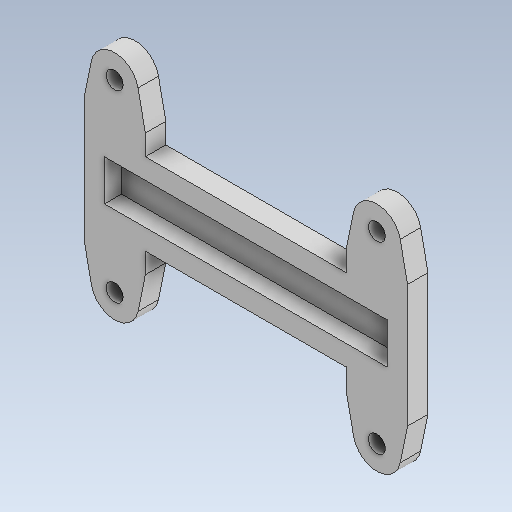
# Autodesk Inventor part: アーム下板
Saved by Autodesk Inventor 2020 (Build 240168000, 168)
## iProperties
Created: 2020-01-11
Part Number: アーム下板
Material: 一般
Document SubType Name: Modeling
Designer: tanjihayato
Density: 1 g/cm^3
Appearance: 既定
Mass: 2.01957 g
Surface Area: 26.5627 cm^2
Volume: 2.01957 cm^3
Author: tanjihayato
Autodesk Inventor part; units mm, degrees
ref_plane "YZ Plane" through (0, 0, 0) normal (1, 0, 0) x (0, 1, 0)
ref_plane "XZ Plane" through (0, 0, 0) normal (0, 1, 0) x (-1, 0, 0)
ref_plane "XY Plane" through (0, 0, 0) normal (0, 0, 1) x (1, 0, 0)
sketch "スケッチ1" plane through (0, 0, 0) normal (0, 0, 1) x (1, 0, 0)
  circle A0 centre (50.4, -4.5) radius 1.5
  circle A1 centre (50.4, -59) radius 1.5
  circle A2 centre (50.4, -86) radius 1.5
  circle A3 centre (50.4, -173.5) radius 1.5
  circle A4 centre (30.9, -4.5) radius 1.5
  circle A5 centre (30.9, -173.5) radius 1.5
  circle A6 centre (75.4, -4.5) radius 1.5
  circle A7 centre (75.4, -173.5) radius 1.5
  line L0 (38.1151, -78.5) -> (38.1151, -81.5)
  arc A8 (36.0151, -81.5) -> (38.1151, -81.5) centre (37.0651, -81.5) ccw
  line L1 (36.0151, -81.5) -> (25.2151, -81.5)
  arc A9 (23.1151, -81.5) -> (25.2151, -81.5) centre (24.1651, -81.5) ccw
  line L2 (23.1151, -81.5) -> (23.1151, -78.5)
  arc A10 (25.2151, -78.5) -> (23.1151, -78.5) centre (24.1651, -78.5) ccw
  line L3 (25.2151, -78.5) -> (36.0151, -78.5)
  arc A11 (38.1151, -78.5) -> (36.0151, -78.5) centre (37.0651, -78.5) ccw
  line L4 (-15.3701, -66.5) -> (-15.3701, -63.5)
  arc A12 (-13.2701, -63.5) -> (-15.3701, -63.5) centre (-14.3201, -63.5) ccw
  line L5 (-13.2701, -63.5) -> (-2.4701, -63.5)
  arc A13 (-0.3701, -63.5) -> (-2.4701, -63.5) centre (-1.4201, -63.5) ccw
  line L6 (-0.3701, -63.5) -> (-0.3701, -66.5)
  arc A14 (-2.4701, -66.5) -> (-0.3701, -66.5) centre (-1.4201, -66.5) ccw
  line L7 (-2.4701, -66.5) -> (-13.2701, -66.5)
  arc A15 (-15.3701, -66.5) -> (-13.2701, -66.5) centre (-14.3201, -66.5) ccw
  line L8 (-0.3701, -78.5) -> (-0.3701, -81.5)
  arc A16 (-2.4701, -81.5) -> (-0.3701, -81.5) centre (-1.4201, -81.5) ccw
  line L9 (-2.4701, -81.5) -> (-13.2701, -81.5)
  arc A17 (-15.3701, -81.5) -> (-13.2701, -81.5) centre (-14.3201, -81.5) ccw
  line L10 (-15.3701, -81.5) -> (-15.3701, -78.5)
  arc A18 (-13.2701, -78.5) -> (-15.3701, -78.5) centre (-14.3201, -78.5) ccw
  line L11 (-13.2701, -78.5) -> (-2.4701, -78.5)
  arc A19 (-0.3701, -78.5) -> (-2.4701, -78.5) centre (-1.4201, -78.5) ccw
  line L12 (23.1151, -66.5) -> (23.1151, -63.5)
  arc A20 (25.2151, -63.5) -> (23.1151, -63.5) centre (24.1651, -63.5) ccw
  line L13 (25.2151, -63.5) -> (36.0151, -63.5)
  arc A21 (38.1151, -63.5) -> (36.0151, -63.5) centre (37.0651, -63.5) ccw
  line L14 (38.1151, -63.5) -> (38.1151, -66.5)
  arc A22 (36.0151, -66.5) -> (38.1151, -66.5) centre (37.0651, -66.5) ccw
  line L15 (36.0151, -66.5) -> (25.2151, -66.5)
  arc A23 (23.1151, -66.5) -> (25.2151, -66.5) centre (24.1651, -66.5) ccw
  line L16 (-108.585, -50) -> (-111.585, -50)
  line L17 (-111.585, -50) -> (-111.585, -128)
  line L18 (-111.585, -128) -> (-108.585, -128)
  arc A24 (-108.585, -130.1) -> (-108.585, -128) centre (-108.585, -129.05) ccw
  line L19 (-108.585, -130.1) -> (-108.585, -140.9)
  arc A25 (-108.585, -143) -> (-108.585, -140.9) centre (-108.585, -141.95) ccw
  line L20 (-108.585, -143) -> (-111.585, -143)
  line L21 (-111.585, -143) -> (-111.585, -168)
  line L22 (-111.585, -168) -> (-108.585, -168)
  line L23 (-108.585, -168) -> (-108.585, -165)
  arc A26 (-106.485, -165) -> (-108.585, -165) centre (-107.535, -165) ccw
  line L24 (-106.485, -165) -> (-95.685, -165)
  arc A27 (-93.585, -165) -> (-95.685, -165) centre (-94.635, -165) ccw
  line L25 (-93.585, -165) -> (-93.585, -168)
  line L26 (-93.585, -168) -> (-20.5995, -168)
  line L27 (-20.5995, -168) -> (-20.5995, -165)
  arc A28 (-18.4995, -165) -> (-20.5995, -165) centre (-19.5495, -165) ccw
  line L28 (-18.4995, -165) -> (-7.6995, -165)
  arc A29 (-5.5995, -165) -> (-7.6995, -165) centre (-6.6495, -165) ccw
  line L29 (-5.5995, -165) -> (-5.5995, -168)
  line L30 (-5.5995, -168) -> (21.4, -168)
  arc A30 (26.4, -173) -> (21.4, -168) centre (21.4, -173) ccw
  line L31 (26.4, -173) -> (26.4, -178)
  line L32 (26.4, -178) -> (40.3, -178)
  arc A31 (42.4, -178) -> (40.3, -178) centre (41.35, -178) ccw
  line L33 (42.4, -178) -> (42.4, -181)
  line L34 (42.4, -181) -> (67.4, -181)
  line L35 (67.4, -181) -> (67.4, -178)
  arc A32 (69.5, -178) -> (67.4, -178) centre (68.45, -178) ccw
  line L36 (69.5, -178) -> (79.9, -178)
  line L37 (79.9, -178) -> (79.9, -164.3045)
  line L38 (79.9, -164.3045) -> (54.9, -129)
  line L39 (54.9, -129) -> (54.9, -49)
  line L40 (54.9, -49) -> (79.9, -13.6955)
  line L41 (79.9, -13.6955) -> (79.9, 0)
  line L42 (79.9, 0) -> (69.5, 0)
  arc A33 (67.4, 0) -> (69.5, 0) centre (68.45, 0) ccw
  line L43 (67.4, 0) -> (67.4, 3)
  line L44 (67.4, 3) -> (42.4, 3)
  line L45 (42.4, 3) -> (42.4, 0)
  arc A34 (40.3, 0) -> (42.4, 0) centre (41.35, 0) ccw
  line L46 (40.3, 0) -> (26.4, 0)
  line L47 (26.4, 0) -> (26.4, -5)
  arc A35 (21.4, -10) -> (26.4, -5) centre (21.4, -5) ccw
  line L48 (21.4, -10) -> (-5.5995, -10)
  line L49 (-5.5995, -10) -> (-5.5995, -13)
  arc A36 (-7.6995, -13) -> (-5.5995, -13) centre (-6.6495, -13) ccw
  line L50 (-7.6995, -13) -> (-18.4995, -13)
  arc A37 (-20.5995, -13) -> (-18.4995, -13) centre (-19.5495, -13) ccw
  line L51 (-20.5995, -13) -> (-20.5995, -10)
  line L52 (-20.5995, -10) -> (-93.585, -10)
  line L53 (-93.585, -10) -> (-93.585, -13)
  arc A38 (-95.685, -13) -> (-93.585, -13) centre (-94.635, -13) ccw
  line L54 (-95.685, -13) -> (-106.485, -13)
  arc A39 (-108.585, -13) -> (-106.485, -13) centre (-107.535, -13) ccw
  line L55 (-108.585, -13) -> (-108.585, -10)
  line L56 (-108.585, -10) -> (-111.585, -10)
  line L57 (-111.585, -10) -> (-111.585, -35)
  line L58 (-111.585, -35) -> (-108.585, -35)
  arc A40 (-108.585, -37.1) -> (-108.585, -35) centre (-108.585, -36.05) ccw
  line L59 (-108.585, -37.1) -> (-108.585, -47.9)
  arc A41 (-108.585, -50) -> (-108.585, -47.9) centre (-108.585, -48.95) ccw
  circle A42 centre (-13.0995, -160.5) radius 1.5
  circle A43 centre (-7.8701, -86) radius 1.5
  circle A44 centre (-104.085, -42.5) radius 1.5
  circle A45 centre (-101.085, -17.5) radius 1.5
  circle A46 centre (30.6151, -86) radius 1.5
  circle A47 centre (-101.085, -160.5) radius 1.5
  circle A48 centre (-7.8701, -59) radius 1.5
  circle A49 centre (-13.0995, -17.5) radius 1.5
  circle A50 centre (30.6151, -59) radius 1.5
  circle A51 centre (-104.085, -135.5) radius 1.5
  line L60 (41.7169, -52.0665) -> (40.5915, -53.6558)
  arc A52 (38.9593, -54.5) -> (40.5915, -53.6558) centre (38.9593, -52.5) ccw
  line L61 (38.9593, -54.5) -> (24.9, -54.5)
  arc A53 (22.9, -52.5) -> (24.9, -54.5) centre (24.9, -52.5) ccw
  line L62 (22.9, -52.5) -> (22.9, -23.5284)
  arc A54 (26.6491, -22.5585) -> (22.9, -23.5284) centre (24.9, -23.5284) ccw
  line L63 (26.6491, -22.5585) -> (41.8338, -49.9408)
  arc A55 (41.7169, -52.0665) -> (41.8338, -49.9408) centre (40.0847, -50.9107) ccw
  arc A56 (-15.846, -59.7485) -> (-18.3701, -63.5) centre (-14.3201, -63.5) ccw
  line L64 (-18.3701, -63.5) -> (-18.3701, -66.5)
  arc A57 (-18.3701, -66.5) -> (-15.846, -70.2515) centre (-14.3201, -66.5) ccw
  arc A58 (-14.5995, -72.1042) -> (-15.846, -70.2515) centre (-16.5995, -72.1042) ccw
  line L65 (-14.5995, -72.1042) -> (-14.5995, -72.8958)
  arc A59 (-15.846, -74.7485) -> (-14.5995, -72.8958) centre (-16.5995, -72.8958) ccw
  arc A60 (-15.846, -74.7485) -> (-18.3701, -78.5) centre (-14.3201, -78.5) ccw
  line L66 (-18.3701, -78.5) -> (-18.3701, -81.5)
  arc A61 (-18.3701, -81.5) -> (-17.3586, -84.1777) centre (-14.3201, -81.5) ccw
  arc A62 (-18.8591, -87.5) -> (-17.3586, -84.1777) centre (-18.8591, -85.5) ccw
  line L67 (-18.8591, -87.5) -> (-50.8293, -87.5)
  arc A63 (-52.5327, -84.4519) -> (-50.8293, -87.5) centre (-50.8293, -85.5) ccw
  line L68 (-52.5327, -84.4519) -> (-18.3029, -28.8193)
  arc A64 (-14.5995, -29.8674) -> (-18.3029, -28.8193) centre (-16.5995, -29.8674) ccw
  line L69 (-14.5995, -29.8674) -> (-14.5995, -57.8958)
  arc A65 (-15.846, -59.7485) -> (-14.5995, -57.8958) centre (-16.5995, -57.8958) ccw
  arc A66 (36.4558, -117.8675) -> (36.8236, -119.0233) centre (38.4558, -117.8675) ccw
  line L70 (36.8236, -119.0233) -> (41.7169, -125.9335)
  arc A67 (41.8338, -128.0592) -> (41.7169, -125.9335) centre (40.0847, -127.0893) ccw
  line L71 (41.8338, -128.0592) -> (26.6491, -155.4415)
  arc A68 (22.9, -154.4716) -> (26.6491, -155.4415) centre (24.9, -154.4716) ccw
  line L72 (22.9, -154.4716) -> (22.9, -92.5)
  arc A69 (24.9, -90.5) -> (22.9, -92.5) centre (24.9, -92.5) ccw
  line L73 (24.9, -90.5) -> (34.4558, -90.5)
  arc A70 (36.4558, -92.5) -> (34.4558, -90.5) centre (34.4558, -92.5) ccw
  line L74 (36.4558, -92.5) -> (36.4558, -117.8675)
  line L75 (68.3465, -169) -> (30.9, -169)
  arc A71 (30.9, -169) -> (29.938, -169.104) centre (30.9, -173.5) ccw
  arc A72 (27.8884, -168.3202) -> (29.938, -169.104) centre (29.5105, -167.1502) ccw
  arc A73 (27.8884, -168.3202) -> (26.0095, -166.4614) centre (21.4, -173) ccw
  arc A74 (25.4128, -163.8569) -> (26.0095, -166.4614) centre (27.1618, -164.8268) ccw
  line L76 (25.4128, -163.8569) -> (42.8246, -132.4585)
  arc A75 (46.2058, -132.2726) -> (42.8246, -132.4585) centre (44.5736, -133.4285) ccw
  line L77 (46.2058, -132.2726) -> (69.9787, -165.8442)
  arc A76 (68.3465, -169) -> (69.9787, -165.8442) centre (68.3465, -167) ccw
  line L78 (-18.3029, -149.1807) -> (-52.5327, -93.5481)
  arc A77 (-50.8293, -90.5) -> (-52.5327, -93.5481) centre (-50.8293, -92.5) ccw
  line L79 (-50.8293, -90.5) -> (-16.5995, -90.5)
  arc A78 (-14.5995, -92.5) -> (-16.5995, -90.5) centre (-16.5995, -92.5) ccw
  line L80 (-14.5995, -92.5) -> (-14.5995, -148.1326)
  arc A79 (-18.3029, -149.1807) -> (-14.5995, -148.1326) centre (-16.5995, -148.1326) ccw
  line L81 (42.8246, -45.5415) -> (25.4128, -14.1431)
  arc A80 (26.0095, -11.5386) -> (25.4128, -14.1431) centre (27.1618, -13.1732) ccw
  arc A81 (26.0095, -11.5386) -> (27.8884, -9.6798) centre (21.4, -5) ccw
  arc A82 (29.938, -8.896) -> (27.8884, -9.6798) centre (29.5105, -10.8498) ccw
  arc A83 (29.938, -8.896) -> (30.9, -9) centre (30.9, -4.5) ccw
  line L82 (30.9, -9) -> (68.3465, -9)
  arc A84 (69.9787, -12.1558) -> (68.3465, -9) centre (68.3465, -11) ccw
  line L83 (69.9787, -12.1558) -> (46.2058, -45.7274)
  arc A85 (42.8246, -45.5415) -> (46.2058, -45.7274) centre (44.5736, -44.5715) ccw
  arc A86 (-10.6764, -21.2919) -> (-8.7291, -18.572) centre (-13.0995, -17.5) ccw
  arc A87 (-6.7413, -17.049) -> (-8.7291, -18.572) centre (-6.7866, -19.0484) ccw
  arc A88 (-6.7413, -17.049) -> (-2.8272, -14.3388) centre (-6.6495, -13) ccw
  arc A89 (-0.9396, -13) -> (-2.8272, -14.3388) centre (-0.9396, -15) ccw
  line L84 (-0.9396, -13) -> (17.9, -13)
  arc A90 (19.9, -15) -> (17.9, -13) centre (17.9, -15) ccw
  line L85 (19.9, -15) -> (19.9, -52.5)
  arc A91 (17.9, -54.5) -> (19.9, -52.5) centre (17.9, -52.5) ccw
  line L86 (17.9, -54.5) -> (-9.5995, -54.5)
  arc A92 (-11.5995, -52.5) -> (-9.5995, -54.5) centre (-9.5995, -52.5) ccw
  line L87 (-11.5995, -52.5) -> (-11.5995, -22.9772)
  arc A93 (-10.6764, -21.2919) -> (-11.5995, -22.9772) centre (-9.5995, -22.9772) ccw
  line L88 (-88.9251, -13) -> (-25.2594, -13)
  arc A94 (-23.3718, -14.3388) -> (-25.2594, -13) centre (-25.2594, -15) ccw
  arc A95 (-23.3718, -14.3388) -> (-19.4577, -17.049) centre (-19.5495, -13) ccw
  arc A96 (-17.47, -18.572) -> (-19.4577, -17.049) centre (-19.4124, -19.0484) ccw
  arc A97 (-17.47, -18.572) -> (-17.1503, -19.4598) centre (-13.0995, -17.5) ccw
  arc A98 (-17.2473, -21.3789) -> (-17.1503, -19.4598) centre (-18.9507, -20.3308) ccw
  line L89 (-17.2473, -21.3789) -> (-55.3889, -83.3691)
  arc A99 (-58.7956, -83.3691) -> (-55.3889, -83.3691) centre (-57.0923, -82.3211) ccw
  line L90 (-58.7956, -83.3691) -> (-96.9372, -21.3789)
  arc A100 (-97.0342, -19.4598) -> (-96.9372, -21.3789) centre (-95.2338, -20.3308) ccw
  arc A101 (-97.0342, -19.4598) -> (-96.7146, -18.572) centre (-101.085, -17.5) ccw
  arc A102 (-94.7268, -17.049) -> (-96.7146, -18.572) centre (-94.7721, -19.0484) ccw
  arc A103 (-94.7268, -17.049) -> (-90.8127, -14.3388) centre (-94.635, -13) ccw
  arc A104 (-88.9251, -13) -> (-90.8127, -14.3388) centre (-88.9251, -15) ccw
  line L91 (-9.5995, -90.5) -> (17.9, -90.5)
  arc A105 (19.9, -92.5) -> (17.9, -90.5) centre (17.9, -92.5) ccw
  line L92 (19.9, -92.5) -> (19.9, -163)
  arc A106 (17.9, -165) -> (19.9, -163) centre (17.9, -163) ccw
  line L93 (17.9, -165) -> (-0.9396, -165)
  arc A107 (-2.8272, -163.6612) -> (-0.9396, -165) centre (-0.9396, -163) ccw
  arc A108 (-2.8272, -163.6612) -> (-6.7413, -160.951) centre (-6.6495, -165) ccw
  arc A109 (-8.7291, -159.428) -> (-6.7413, -160.951) centre (-6.7866, -158.9516) ccw
  arc A110 (-8.7291, -159.428) -> (-10.6764, -156.7081) centre (-13.0995, -160.5) ccw
  arc A111 (-11.5995, -155.0228) -> (-10.6764, -156.7081) centre (-9.5995, -155.0228) ccw
  line L94 (-11.5995, -155.0228) -> (-11.5995, -92.5)
  arc A112 (-9.5995, -90.5) -> (-11.5995, -92.5) centre (-9.5995, -92.5) ccw
  arc A113 (-107.2462, -145.7723) -> (-104.536, -141.8582) centre (-108.585, -141.95) ccw
  arc A114 (-103.013, -139.8704) -> (-104.536, -141.8582) centre (-102.5366, -141.8129) ccw
  arc A115 (-103.013, -139.8704) -> (-103.013, -131.1296) centre (-104.085, -135.5) ccw
  arc A116 (-104.536, -129.1418) -> (-103.013, -131.1296) centre (-102.5366, -129.1871) ccw
  arc A117 (-104.536, -129.1418) -> (-107.2462, -125.2277) centre (-108.585, -129.05) ccw
  arc A118 (-108.585, -123.3401) -> (-107.2462, -125.2277) centre (-106.585, -123.3401) ccw
  line L95 (-108.585, -123.3401) -> (-108.585, -92.5)
  arc A119 (-106.585, -90.5) -> (-108.585, -92.5) centre (-106.585, -92.5) ccw
  line L96 (-106.585, -90.5) -> (-63.3552, -90.5)
  arc A120 (-61.6518, -93.5481) -> (-63.3552, -90.5) centre (-63.3552, -92.5) ccw
  line L97 (-61.6518, -93.5481) -> (-99.4923, -155.049)
  arc A121 (-101.1616, -156.0007) -> (-99.4923, -155.049) centre (-101.1957, -154.0009) ccw
  arc A122 (-101.1616, -156.0007) -> (-105.4554, -159.428) centre (-101.085, -160.5) ccw
  arc A123 (-107.4432, -160.951) -> (-105.4554, -159.428) centre (-107.3979, -158.9516) ccw
  arc A124 (-108.585, -159.1445) -> (-107.4432, -160.951) centre (-106.585, -159.1445) ccw
  line L98 (-108.585, -159.1445) -> (-108.585, -147.6599)
  arc A125 (-107.2462, -145.7723) -> (-108.585, -147.6599) centre (-106.585, -147.6599) ccw
  line L99 (-25.2594, -165) -> (-88.9251, -165)
  arc A126 (-90.8127, -163.6612) -> (-88.9251, -165) centre (-88.9251, -163) ccw
  arc A127 (-90.8127, -163.6612) -> (-94.7268, -160.951) centre (-94.635, -165) ccw
  arc A128 (-96.7146, -159.428) -> (-94.7268, -160.951) centre (-94.7721, -158.9516) ccw
  arc A129 (-96.7146, -159.428) -> (-97.0342, -158.5402) centre (-101.085, -160.5) ccw
  arc A130 (-96.9372, -156.6211) -> (-97.0342, -158.5402) centre (-95.2338, -157.6692) ccw
  line L100 (-96.9372, -156.6211) -> (-58.7956, -94.6309)
  arc A131 (-55.3889, -94.6309) -> (-58.7956, -94.6309) centre (-57.0923, -95.6789) ccw
  line L101 (-55.3889, -94.6309) -> (-17.2473, -156.6211)
  arc A132 (-17.1503, -158.5402) -> (-17.2473, -156.6211) centre (-18.9507, -157.6692) ccw
  arc A133 (-17.1503, -158.5402) -> (-17.47, -159.428) centre (-13.0995, -160.5) ccw
  arc A134 (-19.4577, -160.951) -> (-17.47, -159.428) centre (-19.4124, -158.9516) ccw
  arc A135 (-19.4577, -160.951) -> (-23.3718, -163.6612) centre (-19.5495, -165) ccw
  arc A136 (-25.2594, -165) -> (-23.3718, -163.6612) centre (-25.2594, -163) ccw
  line L102 (-4.8263, -75.5) -> (-9.5995, -75.5)
  arc A137 (-11.5995, -73.5) -> (-9.5995, -75.5) centre (-9.5995, -73.5) ccw
  line L103 (-11.5995, -73.5) -> (-11.5995, -71.5)
  arc A138 (-9.5995, -69.5) -> (-11.5995, -71.5) centre (-9.5995, -71.5) ccw
  line L104 (-9.5995, -69.5) -> (-4.8263, -69.5)
  arc A139 (-3.7003, -69.8471) -> (-4.8263, -69.5) centre (-4.8263, -71.5) ccw
  arc A140 (-3.7003, -69.8471) -> (2.4022, -67.8388) centre (-1.4201, -66.5) ccw
  arc A141 (4.2898, -66.5) -> (2.4022, -67.8388) centre (4.2898, -68.5) ccw
  line L105 (4.2898, -66.5) -> (17.9, -66.5)
  arc A142 (19.9, -68.5) -> (17.9, -66.5) centre (17.9, -68.5) ccw
  line L106 (19.9, -68.5) -> (19.9, -76.5)
  arc A143 (17.9, -78.5) -> (19.9, -76.5) centre (17.9, -76.5) ccw
  line L107 (17.9, -78.5) -> (4.2898, -78.5)
  arc A144 (2.4022, -77.1612) -> (4.2898, -78.5) centre (4.2898, -76.5) ccw
  arc A145 (2.4022, -77.1612) -> (-3.7003, -75.1529) centre (-1.4201, -78.5) ccw
  arc A146 (-4.8263, -75.5) -> (-3.7003, -75.1529) centre (-4.8263, -73.5) ccw
  arc A147 (-107.2462, -52.7723) -> (-104.536, -48.8582) centre (-108.585, -48.95) ccw
  arc A148 (-103.013, -46.8704) -> (-104.536, -48.8582) centre (-102.5366, -48.8129) ccw
  arc A149 (-103.013, -46.8704) -> (-103.013, -38.1296) centre (-104.085, -42.5) ccw
  arc A150 (-104.536, -36.1418) -> (-103.013, -38.1296) centre (-102.5366, -36.1871) ccw
  arc A151 (-104.536, -36.1418) -> (-107.2462, -32.2277) centre (-108.585, -36.05) ccw
  arc A152 (-108.585, -30.3401) -> (-107.2462, -32.2277) centre (-106.585, -30.3401) ccw
  line L108 (-108.585, -30.3401) -> (-108.585, -18.9749)
  arc A153 (-106.899, -16.9998) -> (-108.585, -18.9749) centre (-106.585, -18.9749) ccw
  arc A154 (-105.4749, -18.4894) -> (-106.899, -16.9998) centre (-107.426, -18.9291) ccw
  arc A155 (-105.4749, -18.4894) -> (-101.1616, -21.9993) centre (-101.085, -17.5) ccw
  arc A156 (-99.4923, -22.951) -> (-101.1616, -21.9993) centre (-101.1957, -23.9991) ccw
  line L109 (-99.4923, -22.951) -> (-61.6518, -84.4519)
  arc A157 (-63.3552, -87.5) -> (-61.6518, -84.4519) centre (-63.3552, -85.5) ccw
  line L110 (-63.3552, -87.5) -> (-106.585, -87.5)
  arc A158 (-108.585, -85.5) -> (-106.585, -87.5) centre (-106.585, -85.5) ccw
  line L111 (-108.585, -85.5) -> (-108.585, -54.6599)
  arc A159 (-107.2462, -52.7723) -> (-108.585, -54.6599) centre (-106.585, -54.6599) ccw
  line L112 (50.4, -4.5) -> (50.4, -173.5) construction
  line L113 (30.9, -4.5) -> (75.4, -4.5) construction
  line L114 (30.9, -173.5) -> (75.4, -173.5) construction
  line L115 (-7.8701, -86) -> (81.4809, -86) construction
  line L116 (-7.8701, -59) -> (87.5371, -59) construction
  point P0 (0, 0)
  point P1 (0, 0)
  dimension "d0" = 3
  dimension "d1" = 3
  dimension "d2" = 3
  dimension "d3" = 3
  dimension "d4" = 4.5
  constraints: 284 point on circle, 234 end point, 160 centre point, 6 point on line, 4 horizontal, 1 vertical
  measures "d0" diameter of A0
  measures "d1" diameter of A1
  measures "d2" diameter of A2
  measures "d3" diameter of A3
  measures "d4" distance between parallel lines of L39 L112
sketch "スケッチ2" plane through (0, 0, 0) normal (0, 0, 1) x (1, 0, 0)
  circle A0 centre (-7.8701, -59) radius 1.5 construction
  circle A1 centre (30.6151, -59) radius 1.5 construction
  circle A2 centre (30.6151, -86) radius 1.5 construction
  circle A3 centre (-7.8701, -86) radius 1.5 construction
  line L0 (-2.4701, -66.5) -> (-13.2701, -66.5) construction
  line L1 (-13.2701, -78.5) -> (-2.4701, -78.5) construction
  circle A4 centre (-7.8701, -59) radius 1.25
  circle A5 centre (30.6151, -59) radius 1.25
  circle A6 centre (-7.8701, -86) radius 1.25
  circle A7 centre (30.6151, -86) radius 1.25
  arc A8 (-11.2982, -86.7059) -> (-4.442, -86.7059) centre (-7.8701, -86) ccw
  arc A9 (27.187, -86.7059) -> (34.0432, -86.7059) centre (30.6151, -86) ccw
  arc A10 (34.0432, -58.2941) -> (27.187, -58.2941) centre (30.6151, -59) ccw
  arc A11 (-4.442, -58.2941) -> (-11.2982, -58.2941) centre (-7.8701, -59) ccw
  line L2 (-12.3701, -63.5) -> (-12.3701, -81.5)
  line L3 (-12.3701, -81.5) -> (-11.2982, -86.7059)
  line L4 (-12.3701, -63.5) -> (-11.2982, -58.2941)
  line L5 (-4.442, -58.2941) -> (-3.3701, -63.5)
  line L6 (-3.3701, -63.5) -> (-3.3701, -66.5)
  line L7 (-3.3701, -66.5) -> (26.1151, -66.5)
  line L8 (26.1151, -66.5) -> (26.1151, -63.5)
  line L9 (26.1151, -63.5) -> (27.187, -58.2941)
  line L10 (34.0432, -58.2941) -> (35.1151, -63.5)
  line L11 (35.1151, -63.5) -> (35.1151, -81.5)
  line L12 (35.1151, -81.5) -> (34.0432, -86.7059)
  line L13 (27.187, -86.7059) -> (26.1151, -81.5)
  line L14 (26.1151, -81.5) -> (26.1151, -78.5)
  line L15 (26.1151, -78.5) -> (-3.3701, -78.5)
  line L16 (-3.3701, -78.5) -> (-3.3701, -81.5)
  line L17 (-3.3701, -81.5) -> (-4.442, -86.7059)
  point P0 (0, 0)
  dimension "d5" = 2.5
  dimension "d6" = 2.5
  dimension "d7" = 2.5
  dimension "d8" = 2.5
  dimension "d9" = 7
  dimension "d10" = 7
  dimension "d11" = 7
  dimension "d12" = 7
  dimension "d13" = 9
  dimension "d14" = 4.5
  dimension "d15" = 4.5
  dimension "d16" = 9
  dimension "d17" = 3
  dimension "d18" = 3
  dimension "d19" = 3
  dimension "d20" = 3
  dimension "d21" = 3
  constraints: 32 end point, 8 centre point, 8 coincident, 8 point on circle, 8 tangent, 4 parallel, 4 perpendicular, 3 collinear, 3 point on line, 1 vertical
  measures "d5" diameter of A4
  measures "d6" diameter of A5
  measures "d7" diameter of A6
  measures "d8" diameter of A7
  measures "d9" diameter of A8
  measures "d10" diameter of A9
  measures "d11" diameter of A10
  measures "d12" diameter of A11
  measures "d13" distance between parallel lines of L6 L2
  measures "d14" distance from line of L2 A0.centre
  measures "d15" distance from line of A1.centre L11
  measures "d16" distance between parallel lines of L8 L11
  measures "d17" distance of L5.end L6.end
  measures "d18" distance of L7.end L8.end
  measures "d19" distance of L13.end L14.end
  measures "d20" distance of L15.end L16.end
  measures "d21" distance from line of L2.end L15
extrude "押し出し1" add sketch "スケッチ2" along normal blind 3
sketch "スケッチ3" plane through (0, 0, 3) normal (0, 0, 1) x (1, 0, 0)
  arc A0 (-4.442, -58.2941) -> (-11.2982, -58.2941) centre (-7.8701, -59) ccw projected
  line L0 (-11.2982, -58.2941) -> (-12.3701, -63.5) projected
  line L1 (-12.3701, -63.5) -> (-12.3701, -81.5) projected
  line L2 (-12.3701, -81.5) -> (-11.2982, -86.7059) projected
  arc A1 (-11.2982, -86.7059) -> (-4.442, -86.7059) centre (-7.8701, -86) ccw projected
  line L3 (-4.442, -86.7059) -> (-3.3701, -81.5) projected
  line L4 (-3.3701, -81.5) -> (-3.3701, -78.5) projected
  line L5 (-3.3701, -78.5) -> (26.1151, -78.5) projected
  line L6 (26.1151, -78.5) -> (26.1151, -81.5) projected
  line L7 (26.1151, -81.5) -> (27.187, -86.7059) projected
  arc A2 (27.187, -86.7059) -> (34.0432, -86.7059) centre (30.6151, -86) ccw projected
  line L8 (34.0432, -86.7059) -> (35.1151, -81.5) projected
  line L9 (35.1151, -81.5) -> (35.1151, -63.5) projected
  line L10 (35.1151, -63.5) -> (34.0432, -58.2941) projected
  arc A3 (34.0432, -58.2941) -> (27.187, -58.2941) centre (30.6151, -59) ccw projected
  line L11 (27.187, -58.2941) -> (26.1151, -63.5) projected
  line L12 (26.1151, -63.5) -> (26.1151, -66.5) projected
  line L13 (26.1151, -66.5) -> (-3.3701, -66.5) projected
  line L14 (-3.3701, -66.5) -> (-3.3701, -63.5) projected
  line L15 (-3.3701, -63.5) -> (-4.442, -58.2941) projected
  circle A4 centre (-7.8701, -59) radius 1.25 projected
  circle A5 centre (30.6151, -59) radius 1.25 projected
  circle A6 centre (-7.8701, -86) radius 1.25 projected
  circle A7 centre (30.6151, -86) radius 1.25 projected
  line L16 (-9.3701, -69.5) -> (32.1151, -69.5)
  line L17 (32.1151, -69.5) -> (32.1151, -75.5)
  line L18 (32.1151, -75.5) -> (-9.3701, -75.5)
  line L19 (-9.3701, -75.5) -> (-9.3701, -69.5)
  point P0 (0, 0)
  dimension "d24" = 3
  dimension "d25" = 3
  dimension "d26" = 3
  dimension "d27" = 3
  constraints: 8 end point, 2 parallel, 1 horizontal, 1 perpendicular
  measures "d24" distance between parallel lines of L16 L13
  measures "d25" distance between parallel lines of L5 L18
  measures "d26" distance between parallel lines of L9 L17
  measures "d27" distance between parallel lines of L1 L19
extrude "押し出し2" cut sketch "スケッチ3" against normal blind 2.5 contours L16 L17 L18 L19
